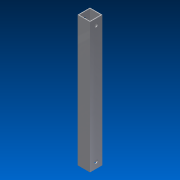
# Autodesk Inventor part: CrossBar
Saved by Autodesk Inventor 2013 (Build 170138000, 138)
## iProperties
Created: 2013-07-23
Part Number: CrossBar
Material: Aluminum 6061
Document SubType Name: Modeling
Designer: orange
Density: 1 g/cm^3
Author: orange
Autodesk Inventor part; units mm, degrees
ref_plane "YZ Plane" through (0, 0, 0) normal (1, 0, 0) x (0, 1, 0)
ref_plane "XZ Plane" through (0, 0, 0) normal (0, 1, 0) x (-1, 0, 0)
ref_plane "XY Plane" through (0, 0, 0) normal (0, 0, 1) x (1, 0, 0)
sketch "Sketch1" plane through (0, 0, 0) normal (0, 1, 0) x (-1, 0, 0)
  line L0 (12.7, 12.7) -> (-12.7, 12.7)
  line L1 (-12.7, 12.7) -> (-12.7, -12.7)
  line L2 (-12.7, -12.7) -> (12.7, -12.7)
  line L3 (12.7, -12.7) -> (12.7, 12.7)
  line L4 (12.7, 12.7) -> (-12.7, -12.7) construction
  line L5 (-12.7, 12.7) -> (12.7, -12.7) construction
  line L6 (-10.9728, -10.9728) -> (10.9728, -10.9728)
  line L7 (10.9728, -10.9728) -> (10.9728, 10.9728)
  line L8 (10.9728, 10.9728) -> (-10.9728, 10.9728)
  line L9 (-10.9728, 10.9728) -> (-10.9728, -10.9728)
  line L10 (-10.9728, -10.9728) -> (10.9728, 10.9728) construction
  line L11 (10.9728, -10.9728) -> (-10.9728, 10.9728) construction
  point P0 (0, 0)
  dimension "d0" = 25.4
  dimension "d2" = 25.4
  dimension "d3" = 1.7272
  constraints: 24 end point, 4 midpoint, 4 parallel, 2 horizontal, 2 perpendicular, 1 point on line
  measures "d0" distance of L1.end L2.end
  measures "d2" distance of L0.end L1.end
  measures "d3" distance between parallel lines of L8 L0
extrude "Extrusion1" add sketch "Sketch1" along normal blind 266.7
sketch "Sketch2" plane through (12.7, 0, 12.7) normal (1, 0, 0) x (0, 0, -1)
  line L0 (0, 0) -> (25.4, 0) projected
  line L1 (25.4, 0) -> (25.4, 266.7) projected
  line L2 (0, 266.7) -> (25.4, 266.7) projected
  line L3 (0, 0) -> (0, 266.7) projected
  point P0 (12.7, 0)
  point P1 (12.7, 254)
  point P2 (12.7, 12.7)
  dimension "d6" = 12.7
  dimension "d7" = 12.7
  dimension "d8" = 12.7
  dimension "d9" = 12.7
  measures "d6" distance from line of L0 point (12.7, 12.7)
  measures "d7" distance from line of L1 point (12.7, 12.7)
  measures "d8" distance from line of point (12.7, 254) L2
  measures "d9" distance from line of L3 point (12.7, 254)
hole "Hole1" at (12.7, 254, 0) at (12.7, 12.7, 0) direction (-1, 0, 0) diameter 6.35 end through all
body "Solid1"
